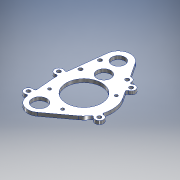
# Autodesk Inventor part: Motor Mount Plate
Saved by Autodesk Inventor 2019.4 (Build 234330000, 330)
## iProperties
Created: 2019-11-30
Part Number: Motor Mount Plate
Material: Aluminum 6061
Document SubType Name: Modeling
Designer: admin
Density: 2.7 g/cm^3
Appearance: Aluminum - Flat
Author: admin
Autodesk Inventor part; units mm, degrees
ref_plane "YZ Plane" through (0, 0, 0) normal (1, 0, 0) x (0, 1, 0)
ref_plane "XZ Plane" through (0, 0, 0) normal (0, 1, 0) x (-1, 0, 0)
ref_plane "XY Plane" through (0, 0, 0) normal (0, 0, 1) x (1, 0, 0)
sketch "Sketch1" plane through (0, 0, 0) normal (0, 1, 0) x (-1, 0, 0)
  circle A0 centre (0, 0) radius 10
  circle A1 centre (11.0348, 81.3072) radius 10 construction
  circle A2 centre (11.0348, 81.3072) radius 10.5
  circle A3 centre (-8.8748, 37.4209) radius 22.3944 construction
  circle A4 centre (-8.8748, 37.4209) radius 25.3944
  circle A5 centre (6.4474, -27.1859) radius 9.5 projected
  arc A6 (0.9094, 94.9628) -> (27.9791, 82.6824) centre (11.0348, 81.3072) ccw construction
  arc A7 (-42.5546, 15.1191) -> (31.2331, 32.6186) centre (-8.8748, 37.4209) ccw construction
  arc A8 (23.8233, -29.2664) -> (-8.1437, -36.8477) centre (6.4474, -27.1859) ccw construction
  line L0 (-8.1437, -36.8477) -> (-42.5546, 15.1191)
  line L1 (23.8233, -29.2664) -> (31.2331, 32.6186)
  line L2 (-32.934, 69.8687) -> (0.9094, 94.9628)
  line L3 (31.3872, 40.6885) -> (27.9791, 82.6824)
  arc A9 (27.9791, 82.6824) -> (0.9094, 94.9628) centre (11.0348, 81.3072) ccw
  arc A10 (-32.934, 69.8687) -> (-42.5546, 15.1191) centre (-8.8748, 37.4209) ccw
  arc A11 (31.3872, 40.6885) -> (-32.934, 69.8687) centre (-8.8748, 37.4209) ccw construction
  arc A12 (31.2331, 32.6186) -> (31.3872, 40.6885) centre (-8.8748, 37.4209) ccw
  arc A13 (-8.1437, -36.8477) -> (23.8233, -29.2664) centre (6.4474, -27.1859) ccw
  dimension "d0" = 20
  dimension "d5" = 0.5
  dimension "d6" = 3
  dimension "d7" = 7
  dimension "d8" = 15
  dimension "d9" = 8
  constraints: 17 point on circle, 15 tangent, 11 centre point, 8 end point, 1 coincident
  measures "d0" diameter of A0
  measures "d5" radial gap between concentric circles of A1 A2
  measures "d6" radial gap between concentric circles of A3 A4
  measures "d7" radial gap between concentric circles of A1 A6
  measures "d8" radial gap between concentric circles of A4 A7
  measures "d9" radial gap between concentric circles of A5 A8
extrude "Extrusion1" add sketch "Sketch1" along normal blind 5
sketch "Sketch2" plane through (0, 0, 0) normal (0, -1, 0) x (1, 0, 0)
  circle A0 centre (35.2337, 17.429) radius 2.2
  circle A1 centre (-20.9595, 57.0259) radius 2.2
  circle A2 centre (13.6085, 72.7436) radius 2.2
  point P0 (0, 0)
  dimension "d12" = 4.4
  dimension "d13" = 4.4
  dimension "d14" = 4.4
  constraints: 3 centre point
  measures "d12" diameter of A0
  measures "d13" diameter of A2
  measures "d14" diameter of A1
extrude "Extrusion2" cut sketch "Sketch2" against normal blind 5
sketch "Sketch3" plane through (0, 0, 0) normal (0, -1, 0) x (1, 0, 0)
  circle A0 centre (35.893, -3.2614) radius 2.75
  circle A1 centre (35.893, -3.2614) radius 6
  circle A2 centre (49.8895, 56.3777) radius 2.75
  circle A3 centre (49.8895, 56.3777) radius 6
  circle A4 centre (-36.0964, 28.5483) radius 2.75
  circle A5 centre (-36.0964, 28.5483) radius 6
  circle A6 centre (-33.3464, 74.8865) radius 2.75
  circle A7 centre (-33.3464, 74.8865) radius 6
  point P0 (0, 0)
  dimension "d18" = 5.5
  dimension "d19" = 12
  dimension "d20" = 5.5
  dimension "d21" = 12
  dimension "d22" = 5.5
  dimension "d23" = 12
  dimension "d24" = 5.5
  dimension "d25" = 12
  constraints: 8 centre point, 4 coincident
  measures "d18" diameter of A0
  measures "d19" diameter of A1
  measures "d20" diameter of A2
  measures "d21" diameter of A3
  measures "d22" diameter of A4
  measures "d23" diameter of A5
  measures "d24" diameter of A6
  measures "d25" diameter of A7
extrude "Extrusion3" add sketch "Sketch3" against normal blind 5
fillet "Fillet1" radius 2 8 edges at (34.194, 2.5, 2.4931) (29.9319, 2.5, -3.9435) (46.8433, 2.5, 51.2085) (43.9784, 2.5, 57.4069) (-28.9425, 2.5, 70.8115) (-28.343, 2.5, 78.198) (-30.4899, 2.5, 26.4113) (-31.1529, 2.5, 31.9486)
sketch "Sketch4" plane through (0, 0, 0) normal (0, -1, 0) x (1, 0, 0)
  circle A0 centre (23.213, -10.311) radius 2.413 projected
  circle A1 centre (-23.213, 10.311) radius 2.413 projected
  circle A2 centre (-20.5361, -14.9476) radius 2.413 projected
  circle A3 centre (23.213, -10.311) radius 2.75
  circle A4 centre (-23.213, 10.311) radius 2.75
  circle A5 centre (-20.5361, -14.9476) radius 2.75
  point P0 (0, 0)
  dimension "d29" = 5.5
  dimension "d30" = 5.5
  dimension "d31" = 5.5
  constraints: 3 centre point, 3 coincident
  measures "d29" diameter of A3
  measures "d30" diameter of A4
  measures "d31" diameter of A5
extrude "Extrusion4" cut sketch "Sketch4" against normal through all contours A0 | A1 | A2 | A3 | A4 | A5
sketch "Sketch5" plane through (0, 0, 0) normal (0, -1, 0) x (1, 0, 0)
  arc A0 (25.9417, -9.9694) -> (23.9637, -12.9565) centre (23.213, -10.311) ccw projected
  circle A1 centre (23.213, -10.311) radius 2.75
  circle A2 centre (23.213, -10.311) radius 6
  point P0 (0, 0)
  dimension "d34" = 12
  constraints: 2 coincident, 1 centre point, 3 other
  measures "d34" diameter of A2
extrude "Extrusion5" add sketch "Sketch5" against normal blind 5
fillet "Fillet2" radius 2 2 edges at (28.0734, 2.5, -6.7929) (21.8469, 2.5, -16.1534)
body "Solid1"
